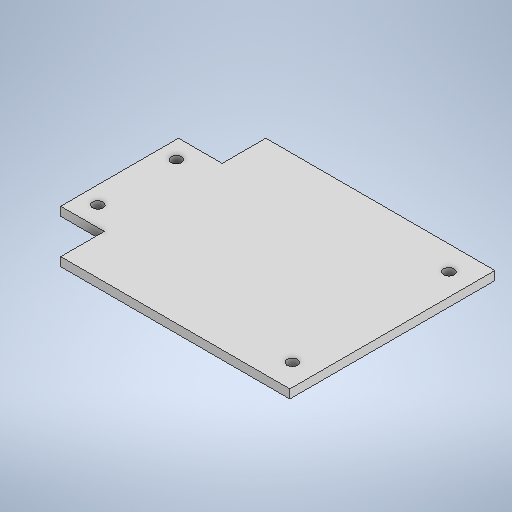
# Autodesk Inventor part: 1.5_base
Saved by Autodesk Inventor 2025 (Build 290162010, 162A)
## iProperties
Created: 2024-05-22
Part Number: 1.5_base
Material: Generic
Document SubType Name: Modeling
Designer: Garfieldcmix
Density: 1 g/cm^3
Appearance: Default
Author: Garfieldcmix
Autodesk Inventor part; units mm, degrees
ref_plane "YZ Plane" through (0, 0, 0) normal (1, 0, 0) x (0, 1, 0)
ref_plane "XZ Plane" through (0, 0, 0) normal (0, 1, 0) x (-1, 0, 0)
ref_plane "XY Plane" through (0, 0, 0) normal (0, 0, 1) x (1, 0, 0)
sketch "Base" plane through (0, 0, 0) normal (0, 1, 0) x (-1, 0, 0)
  line L0 (105, -32) -> (105, -52)
  line L1 (105, -52) -> (125, -52)
  line L2 (105, -32) -> (0, -32)
  line L3 (0, -32) -> (0, -126)
  line L4 (0, -126) -> (105, -126)
  line L5 (105, -126) -> (105, -106)
  line L6 (105, -106) -> (125, -106)
  line L7 (125, -106) -> (125, -52)
  circle A0 centre (117, -61) radius 2.4
  circle A1 centre (117, -97) radius 2.4
  circle A2 centre (10, -43.1) radius 2.4
  circle A3 centre (10, -114.9) radius 2.4
  point P0 (0, 0)
  dimension "d27" = 20
  dimension "d36" = 94
  dimension "d37" = 20
  dimension "d41" = 20
  dimension "d42" = 32
  dimension "d57" = 105
  dimension "d58" = 54
  dimension "d59" = 125
  dimension "d60" = 4.8
  dimension "d61" = 12
  dimension "d62" = 9
  dimension "d63" = 4.8
  dimension "d64" = 12
  dimension "d65" = 9
  dimension "d66" = 4.8
  dimension "d67" = 10
  dimension "d68" = 11.1
  dimension "d69" = 4.8
  dimension "d70" = 11.1
  dimension "d71" = 10
  constraints: 16 end point, 4 centre point, 3 horizontal, 3 perpendicular, 2 vertical, 1 collinear, 1 point on line
  measures "d27" distance of L0.start L0.end
  measures "d36" distance of L2.end L3.end
  measures "d37" distance of L4.end L5.end
  measures "d41" distance between parallel lines of L0 L7
  measures "d42" distance from line of point (0, 0) L2
  measures "d57" distance between parallel lines of L3 L0
  measures "d58" distance from line of L6 L1.end
  measures "d59" distance between parallel lines of L3 L7
  measures "d60" diameter of A0
  measures "d61" horizontal distance of L0.end A0.centre
  measures "d62" distance from line of L1 A0.centre
  measures "d63" diameter of A1
  measures "d64" horizontal distance of L5.end A1.centre
  measures "d65" distance from line of L6 A1.centre
  measures "d66" diameter of A2
  measures "d67" distance from line of L3 A2.centre
  measures "d68" distance from line of L2 A2.centre
  measures "d69" diameter of A3
  measures "d70" distance from line of L4 A3.centre
  measures "d71" distance from line of L3 A3.centre
extrude "Extrusion1" add sketch "Base" along normal blind 4
body "Solid1"
